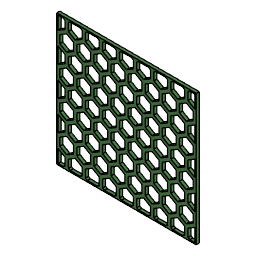
Rig (Autodesk Fusion 360 archive; units mm, degrees)
design "honey comb v1"
Autodesk Fusion 360 part; units mm, degrees
sketch "Sketch2" plane through (0, 0, 0) normal (0, 1, 0) x (1, 0, 0)
  line L0 (10, 5.7735) -> (0, 11.547)
  line L1 (0, 11.547) -> (-10, 5.7735)
  line L2 (-10, 5.7735) -> (-10, -5.7735)
  line L3 (-10, -5.7735) -> (0, -11.547)
  line L4 (0, -11.547) -> (10, -5.7735)
  line L5 (10, -5.7735) -> (10, 5.7735)
  line L6 (0, 0) -> (5, -8.6603) construction
  line L7 (-100, -94) -> (100, -94)
  line L8 (100, -94) -> (100, 94)
  line L9 (100, 94) -> (-100, 94)
  line L10 (-100, 94) -> (-100, -94)
  line L11 (-102, -96) -> (102, -96)
  line L12 (102, -96) -> (102, 96)
  line L13 (102, 96) -> (-102, 96)
  line L14 (-102, 96) -> (-102, -96)
  line L15 (0, -94) -> (0, -96) construction
  line L16 (100, 0) -> (102, 0) construction
  line L17 (-100, 0) -> (-102, 0) construction
  line L18 (0, 94) -> (0, 96) construction
  line L19 (-100, 0) -> (0, 0) construction
  line L20 (0, 0) -> (100, 0) construction
  dimension "d1" = 20
  dimension "d2" = 2
  dimension "d12" = 188
  dimension "d13" = 200
  constraint coincident L6.start L19.end
  constraint midpoint L4 L6.end
  constraint horizontal L7
  constraint perpendicular L7 L8
  constraint parallel L7 L9
  constraint parallel L8 L10
  constraint horizontal L11
  constraint vertical L12
  constraint horizontal L13
  constraint vertical L14
  constraint midpoint L7 L15.start
  constraint coincident L11 L15.end
  constraint perpendicular L11 L15
  constraint midpoint L8 L16.start
  constraint coincident L12 L16.end
  constraint perpendicular L12 L16
  constraint midpoint L10 L17.start
  constraint coincident L14 L17.end
  constraint perpendicular L14 L17
  constraint midpoint L9 L18.start
  constraint coincident L13 L18.end
  constraint perpendicular L13 L18
  constraint equal L15 L17
  constraint equal L17 L18
  constraint equal L16 L18
  constraint perpendicular L2 L19
  constraint perpendicular L8 L20
  constraint equal L19 L20
  measures "d1" distance of L2 L5
  measures "d2" distance of L7 L11
  measures "d12" distance of L7.end L8.end
  measures "d13" distance of L8.end L9.end
extrude "Extrude1" add sketch "Sketch2" against normal blind 10 contours L0 L1 L2 L3 L4 L5 | L7 L8 L9 L10
extrude "Extrude2" cut sketch "Sketch2" against normal through all contours L0 L1 L2 L3 L4 L5
pattern_linear "R-Pattern1" count 19 spacing 25 along (1, 0, 0) both ways count 19 spacing 25 along (0.5, 0, 0.866025) both ways of "Extrude2"
extrude "Extrude3" add sketch "Sketch2" against normal blind 10 contours L11 L12 L13 L14
extrude "Extrude4" cut 1 faces at (-75.8333, -10, -66.8764) along direction (0, 1, 0) blind 5.5
equation "d8 = d1 + 5 mm"
equation "d9 = d1 + 5 mm"

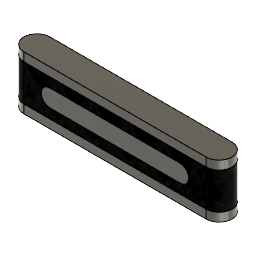
design "Conveyor Belt"
Autodesk Fusion 360 part; units mm, degrees
mirror "Mirror1" [no effect]
sketch "Sketch3" plane through (0, 0, 0) normal (0, 0, 1) x (1, 0, 0)
  line L0 (0, 0) -> (-525, 0)
  line L1 (-525, 0) -> (-525, -75)
  line L2 (-525, -75) -> (0, -75)
  line L3 (0, -75) -> (0, 0)
  circle A0 centre (-525, -37.5) radius 37.5
  circle A1 centre (0, -37.5) radius 37.5
  dimension "d12" = 75
  dimension "d13" = 525
  constraint horizontal L0
  constraint vertical L1
  constraint horizontal L2
  constraint vertical L3
  constraint coincident L0.start L3.end
  constraint coincident L0.end A0
  constraint tangent L0 A0
  constraint coincident L1.end A0
  measures "d12" distance of L0.start L2.end
  measures "d13" distance of L0.start L0.end
extrude "Extrude3" add sketch "Sketch3" along normal blind 155 makes body 1
sketch "Sketch4" plane through (0, -75, 0) normal (0, -1, 0) x (1, 0, 0)
  line L0 (-525, 0) -> (0, 0)
  line L1 (0, 0) -> (0, 155)
  line L2 (0, 155) -> (-525, 155)
  line L3 (-525, 155) -> (-525, 0)
  line L4 (-448.9835, 102.4793) -> (-75.0014, 102.5)
  line L5 (-448.9835, 52.5207) -> (-75.0014, 52.5)
  arc A0 (-448.9835, 102.4793) -> (-448.9835, 52.5207) centre (-450, 77.5) ccw
  arc A1 (-75.0014, 52.5) -> (-75.0014, 102.5) centre (-75, 77.5) ccw
  dimension "d16" = 50
  dimension "d17" = 75
  dimension "d18" = 50
  dimension "d19" = 75
  constraint tangent L4 A1
  constraint tangent L5 A1
  measures "d16" diameter of A0
  measures "d17" distance of L3 A0.centre
  measures "d18" diameter of A1
  measures "d19" distance of L1 A1.centre
extrude "Extrude4" add sketch "Sketch4" along normal blind 0.1 contours L4 L5 A0 A1 bodies 1
extrude "Extrude5" cut 1 faces at (-350, -50, 155) along direction (0, 0, -1) blind 130 on bodies 1 bodies 1 makes body 2 at (-350, -50, 0)
extrude "Extrude6" add 1 faces at (-350, -50, 25) along direction (0, 0, 1) blind 105 separate body on bodies 2 makes body 3
extrude "Extrude7" add 1 faces at (-350, -50, 130) along direction (0, 0, 1) blind 25 separate body on bodies 3 makes body 4
equation "d24 = 130.00 mm - 25 mm"

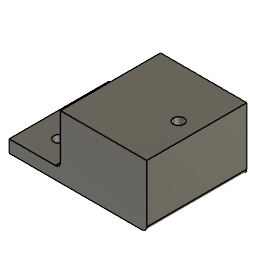
design "Rod Holder Thick"
Autodesk Fusion 360 part; units mm, degrees
sketch "Sketch1" plane through (0, 0, 0) normal (0, 0, 1) x (1, 0, 0)
  line L0 (0, 0) -> (55, 0)
  line L1 (55, 0) -> (55, 40)
  line L2 (55, 40) -> (0, 40)
  line L3 (0, 40) -> (0, 0)
  dimension "d1" = 55
  dimension "d2" = 40
  constraint horizontal L0
  constraint vertical L1
  constraint horizontal L2
  constraint vertical L3
  constraint coincident L0.start L3.end
  measures "d1" distance of L0.start L0.end
  measures "d2" distance of L0.start L2.end
extrude "Extrude1" add sketch "Sketch1" along normal blind 5
sketch "Sketch2" plane through (0, 0, 5) normal (0, 0, 1) x (-1, 0, 0)
  line L0 (0, -40) -> (0, 0)
  line L1 (0, 0) -> (-55, 0)
  line L2 (-55, 0) -> (-55, -40)
  line L3 (-55, -40) -> (0, -40)
  circle A0 centre (-10, -10) radius 2.15
  circle A1 centre (-10, -30) radius 2.15
  circle A2 centre (-47.75, -20) radius 2.15
  line L4 (-20.5, -40) -> (-20.5, 0)
  dimension "d5" = 4.3
  dimension "d6" = 4.3
  dimension "d7" = 20
  dimension "d8" = 10
  dimension "d9" = 10
  dimension "d10" = 4.3
  dimension "d11" = 7.25
  dimension "d12" = 20.5
  constraint coincident L3 L4.start
  constraint coincident L1 L4.end
  constraint perpendicular L1 L4
  measures "d5" diameter of A0
  measures "d6" diameter of A1
  measures "d7" distance of A0.centre A1.centre
  measures "d8" distance of L1 A0.centre
  measures "d9" distance of L0 A0.centre
  measures "d10" diameter of A2
  measures "d11" distance of L2 A2.centre
  measures "d12" distance of L0 L4
extrude "Extrude2" cut sketch "Sketch2" against normal blind 22 contours A0 | A1 | A2
extrude "Extrude3" add sketch "Sketch2" along normal blind 20 contours L1 L2 L3 L4
fillet "Fillet1" radius 2 1 edges at (20.5, 20, 5)
fillet "Fillet2" radius 2 1 edges at (55, 20, 0)

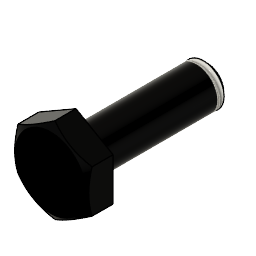
design "Hexagon Head Bolt DIN EN 24014 - M4 x 12 Steel 4.6 Black"
description: Hexagon Head Bolt DIN EN 24014 - M4 x 12
part number: DIN EN 24014 - M4 x 12 Steel 4.6 Black
Autodesk Fusion 360 part; units mm, degrees
sketch "Sketch1" plane through (0, 0, 0) normal (0, 1, 0) x (1, 0, 0)
  line L0 (-2, 0) -> (-2, 12)
  line L1 (-2, 12) -> (0, 12)
  line L2 (0, 12) -> (0, -2.8)
  line L3 (-2.94, -0.4) -> (-4.0425, -0.4)
  line L4 (-4.0425, -0.4) -> (-4.0425, -2.3858)
  line L5 (-2.94, -0.4) -> (-2.7091, 0)
  line L6 (-2.7091, 0) -> (-2, 0)
  line L7 (0, -2.8) -> (-3.325, -2.8)
  line L8 (-4.0425, -2.3858) -> (-3.325, -2.8)
  dimension "d81" = 8.085
  dimension "d123" = 0.4
  dimension "d127" = 12
  dimension "d149" = 4
  dimension "d157" = 30
  dimension "d158" = 6.65
  dimension "d162" = 2.8
  dimension "d163" = 30
  dimension "d164" = 5.88
  constraint perpendicular L0 L1
  constraint vertical L2
  constraint parallel L2 L4
  constraint coincident L2 L7.start
  constraint coincident origin L6
  constraint coincident L0.end L1.start
  constraint perpendicular L2 L7
  constraint coincident origin L2
  measures "d123" distance of L3 L6
  measures "d127" distance of L1 L6
  measures "d157" angle of L7 L8
  measures "d162" distance of L6 L7
  measures "d163" angle of L4 L5
revolve "Revolve1" add sketch "Sketch1" angle 360 about axis through (0, 0, -12) along (0, 0, 1)
sketch "Sketch8" plane through (0, 0, 0) normal (0, 0, 1) x (1, 0, 0)
  circle A0 centre (0, 0) radius 4.0425
  circle A1 centre (0, 0) radius 4.0425
  line L0 (-3.5009, -2.0213) -> (0, -4.0425)
  line L1 (0, -4.0425) -> (3.5009, -2.0212)
  line L2 (3.5009, -2.0212) -> (3.5009, 2.0213)
  line L3 (3.5009, 2.0213) -> (0, 4.0425)
  line L4 (0, 4.0425) -> (-3.5009, 2.0212)
  line L5 (-3.5009, 2.0212) -> (-3.5009, -2.0213)
  constraint coincident A1 L0.start
  constraint coincident A0.centre A1.centre
  constraint vertical L5
extrude "Extrude5" cut sketch "Sketch8" along normal through all contours A0 A1 L2 | A0 A1 L3 | A0 A1 L1 | A0 A1 L4 | A0 A1 L0 | A0 A1 L5
thread "Thread2" "ISO Metric profile 4.0 M4x0.7 M4x0.7 6g" major diameter 3.908 minor diameter 3.111 pitch 0.7 angle 60 resizes the face on face at (-1.9975, 0.0997, -8) from (0, 0, -11) to (0, 0, -12)
fillet "Fillet6" radius 0.2 1 edges at (1.954, 0, 0)
sketch "Sketch15" plane through (0, 0, 0) normal (0, 1, 0) x (1, 0, 0)
  line L0 (-2.04, 12) -> (-2.04, 11.5706)
  line L1 (-2.04, 11.5706) -> (-1.5706, 12)
  line L2 (0, 12) -> (0, -2.8)
  line L3 (-2.04, 12) -> (0, 12)
  dimension "d165" = 1.5706
  dimension "d166" = 2.04
  dimension "d167" = 0.4294
  constraint coincident L2.start L3.end
  constraint perpendicular L2 L3
  constraint coincident L1.end L3
  constraint perpendicular L0 L3
  measures "d165" distance of L1.end L2
  measures "d166" distance of L0 L2.start
  measures "d167" distance of L0.end L3
revolve "Revolve4" cut sketch "Sketch15" angle 360 about axis through (0, 0, 1.75) along (0, 0, 1)
equation "adsk_nomlen = 12.00 mm"
equation "adsk_headh = 2.80 mm"
equation "adsk_headdia = 8.085 mm"
equation "adsk_nomdia = 4.00 mm"
equation "d81 = adsk_headdia"
equation "adsk_waflat = 7.00 mm"
equation "adsk_thrlen = 1.00 mm"
equation "adsk_chamang2 = 30.00 deg"
equation "adsk_midfillet = 0.20 mm"
equation "d123 = adsk_necklen"
equation "adsk_necklen = 0.40 mm"
equation "adsk_neckdia = 5.88 mm"
equation "d127 = adsk_nomlen"
equation "d138 = adsk_midfillet"
equation "d140 = min(adsk_thrlen; adsk_nomlen - adsk_midfillet - 0.01 mm)"
equation "adsk_endpointdia = 3.14117 mm"
equation "adsk_startlen = 0.429415 mm"
equation "d149 = adsk_nomdia"
equation "d157 = adsk_chamang2"
equation "d158 = adsk_waflat * 0.95"
equation "adsk_neckang = 30 deg"
equation "d162 = adsk_headh"
equation "d163 = adsk_neckang"
equation "d164 = adsk_neckdia"
equation "d165 = adsk_endpointdia / 2"
equation "d166 = adsk_nomdia * 0.51"
equation "d167 = adsk_startlen"

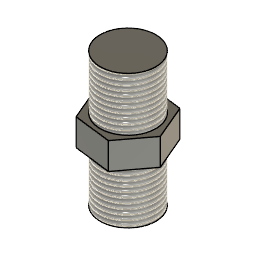
design "Male-Male Adaptor BSP"
Autodesk Fusion 360 part; units mm, degrees
sketch "Sketch1" plane through (0, 0, 0) normal (0, 0, 1) x (1, 0, 0)
  circle A0 centre (0, 0) radius 10
  dimension "d1" = 20
  constraint coincident A0.centre origin
  measures "d1" diameter of A0
extrude "Extrude1" add sketch "Sketch1" along normal blind 20
sketch "Sketch2" plane through (0, 0, 20) normal (0, 0, 1) x (-1, 0, 0)
  circle A0 centre (0, 0) radius 10
  line L0 (-8.3368, -11.0679) -> (5.4167, -12.7538)
  line L1 (5.4167, -12.7538) -> (13.7535, -1.6859)
  line L2 (13.7535, -1.6859) -> (8.3368, 11.0679)
  line L3 (8.3368, 11.0679) -> (-5.4167, 12.7538)
  line L4 (-5.4167, 12.7538) -> (-13.7535, 1.6859)
  line L5 (-13.7535, 1.6859) -> (-8.3368, -11.0679)
  dimension "d4" = 12
  constraint coincident A0.centre origin
  measures "d4" distance of A0.centre L5
extrude "Extrude2" add sketch "Sketch2" along normal blind 10 contours A0 | L0 L1 L2 L3 L4 L5
sketch "Sketch3" plane through (0, 0, 30) normal (0, 0, 1) x (-1, 0, 0)
  line L0 (-13.7535, 1.6859) -> (-8.3368, -11.0679)
  line L1 (-8.3368, -11.0679) -> (5.4167, -12.7538)
  line L2 (5.4167, -12.7538) -> (13.7535, -1.6859)
  line L3 (13.7535, -1.6859) -> (8.3368, 11.0679)
  line L4 (8.3368, 11.0679) -> (-5.4167, 12.7538)
  line L5 (-5.4167, 12.7538) -> (-13.7535, 1.6859)
  circle A0 centre (0, 0) radius 10
  dimension "d7" = 20
  constraint coincident A0.centre origin
  measures "d7" diameter of A0
extrude "Extrude3" add sketch "Sketch3" along normal blind 20 contours A0
thread "Thread1" "BSP Pipe Threads 1/2 G 1/2-14 G 1/2-14" major diameter 20.813 minor diameter 18.631 pitch 1.8143 angle 55 resizes the face on face at (9.9876, -0.4985, 13.3333) on face at (-9.9876, 0.4985, 43.3333)

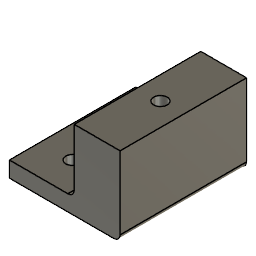
design "Rod Holding Bracket"
Autodesk Fusion 360 part; units mm, degrees
sketch "Sketch1" plane through (0, 0, 0) normal (0, 0, 1) x (1, 0, 0)
  line L0 (0, 0) -> (35, 0)
  line L1 (35, 0) -> (35, 40)
  line L2 (35, 40) -> (0, 40)
  line L3 (0, 40) -> (0, 0)
  dimension "d1" = 35
  dimension "d2" = 40
  constraint horizontal L0
  constraint vertical L1
  constraint horizontal L2
  constraint vertical L3
  constraint coincident L0.start L3.end
  measures "d1" distance of L0.start L0.end
  measures "d2" distance of L0.start L2.end
extrude "Extrude1" add sketch "Sketch1" along normal blind 5
sketch "Sketch2" plane through (0, 0, 5) normal (0, 0, 1) x (-1, 0, 0)
  line L0 (0, -40) -> (0, 0)
  line L1 (0, 0) -> (-35, 0)
  line L2 (-35, 0) -> (-35, -40)
  line L3 (-35, -40) -> (0, -40)
  circle A0 centre (-10, -10) radius 2.15
  circle A1 centre (-10, -30) radius 2.15
  circle A2 centre (-27.75, -20) radius 2.15
  line L4 (-20.5, -40) -> (-20.5, 0)
  dimension "d5" = 4.3
  dimension "d6" = 4.3
  dimension "d7" = 20
  dimension "d8" = 10
  dimension "d9" = 10
  dimension "d10" = 4.3
  dimension "d11" = 7.25
  dimension "d12" = 20.5
  constraint coincident L3 L4.start
  constraint coincident L1 L4.end
  constraint perpendicular L1 L4
  measures "d5" diameter of A0
  measures "d6" diameter of A1
  measures "d7" distance of A0.centre A1.centre
  measures "d8" distance of L1 A0.centre
  measures "d9" distance of L0 A0.centre
  measures "d10" diameter of A2
  measures "d11" distance of L2 A2.centre
  measures "d12" distance of L0 L4
extrude "Extrude2" cut sketch "Sketch2" against normal blind 22 contours A0 | A1 | A2
extrude "Extrude3" add sketch "Sketch2" along normal blind 20 contours L1 L2 L3 L4
fillet "Fillet1" radius 2 1 edges at (20.5, 20, 5)
fillet "Fillet2" radius 2 1 edges at (35, 20, 0)

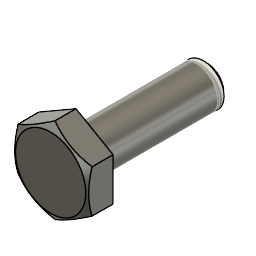
design "Hexagon Head Bolt DIN EN 24014 - M4 x 12 Steel 4.6 Plain"
description: Hexagon Head Bolt DIN EN 24014 - M4 x 12
part number: DIN EN 24014 - M4 x 12 Steel 4.6 Plain
Autodesk Fusion 360 part; units mm, degrees
sketch "Sketch1" plane through (0, 0, 0) normal (0, 1, 0) x (1, 0, 0)
  line L0 (-2, 0) -> (-2, 12)
  line L1 (-2, 12) -> (0, 12)
  line L2 (0, 12) -> (0, -2.8)
  line L3 (-2.94, -0.4) -> (-4.0425, -0.4)
  line L4 (-4.0425, -0.4) -> (-4.0425, -2.3858)
  line L5 (-2.94, -0.4) -> (-2.7091, 0)
  line L6 (-2.7091, 0) -> (-2, 0)
  line L7 (0, -2.8) -> (-3.325, -2.8)
  line L8 (-4.0425, -2.3858) -> (-3.325, -2.8)
  dimension "d81" = 8.085
  dimension "d123" = 0.4
  dimension "d127" = 12
  dimension "d149" = 4
  dimension "d157" = 30
  dimension "d158" = 6.65
  dimension "d162" = 2.8
  dimension "d163" = 30
  dimension "d164" = 5.88
  constraint perpendicular L0 L1
  constraint vertical L2
  constraint parallel L2 L4
  constraint coincident L2 L7.start
  constraint coincident origin L6
  constraint coincident L0.end L1.start
  constraint perpendicular L2 L7
  constraint coincident origin L2
  measures "d123" distance of L3 L6
  measures "d127" distance of L1 L6
  measures "d157" angle of L7 L8
  measures "d162" distance of L6 L7
  measures "d163" angle of L4 L5
revolve "Revolve1" add sketch "Sketch1" angle 360 about axis through (0, 0, -12) along (0, 0, 1)
sketch "Sketch8" plane through (0, 0, 0) normal (0, 0, 1) x (1, 0, 0)
  circle A0 centre (0, 0) radius 4.0425
  circle A1 centre (0, 0) radius 4.0425
  line L0 (-3.5009, -2.0213) -> (0, -4.0425)
  line L1 (0, -4.0425) -> (3.5009, -2.0212)
  line L2 (3.5009, -2.0212) -> (3.5009, 2.0213)
  line L3 (3.5009, 2.0213) -> (0, 4.0425)
  line L4 (0, 4.0425) -> (-3.5009, 2.0212)
  line L5 (-3.5009, 2.0212) -> (-3.5009, -2.0213)
  constraint coincident A1 L0.start
  constraint coincident A0.centre A1.centre
  constraint vertical L5
extrude "Extrude5" cut sketch "Sketch8" along normal through all contours A0 A1 L2 | A0 A1 L3 | A0 A1 L1 | A0 A1 L4 | A0 A1 L0 | A0 A1 L5
thread "Thread2" "ISO Metric profile 4.0 M4x0.7 M4x0.7 6g" major diameter 3.908 minor diameter 3.111 pitch 0.7 angle 60 resizes the face on face at (-1.9901, 0.1991, -8) from (0, 0, -11) to (0, 0, -12)
fillet "Fillet6" radius 0.2 1 edges at (1.954, 0, 0)
sketch "Sketch15" plane through (0, 0, 0) normal (0, 1, 0) x (1, 0, 0)
  line L0 (-2.04, 12) -> (-2.04, 11.5706)
  line L1 (-2.04, 11.5706) -> (-1.5706, 12)
  line L2 (0, 12) -> (0, -2.8)
  line L3 (-2.04, 12) -> (0, 12)
  dimension "d165" = 1.5706
  dimension "d166" = 2.04
  dimension "d167" = 0.4294
  constraint coincident L2.start L3.end
  constraint perpendicular L2 L3
  constraint coincident L1.end L3
  constraint perpendicular L0 L3
  measures "d165" distance of L1.end L2
  measures "d166" distance of L0 L2.start
  measures "d167" distance of L0.end L3
revolve "Revolve4" cut sketch "Sketch15" angle 360 about axis through (0, 0, 1.75) along (0, 0, 1)
equation "adsk_nomlen = 12.00 mm"
equation "adsk_headh = 2.80 mm"
equation "adsk_headdia = 8.085 mm"
equation "adsk_nomdia = 4.00 mm"
equation "d81 = adsk_headdia"
equation "adsk_waflat = 7.00 mm"
equation "adsk_thrlen = 1.00 mm"
equation "adsk_chamang2 = 30.00 deg"
equation "adsk_midfillet = 0.20 mm"
equation "d123 = adsk_necklen"
equation "adsk_necklen = 0.40 mm"
equation "adsk_neckdia = 5.88 mm"
equation "d127 = adsk_nomlen"
equation "d138 = adsk_midfillet"
equation "d140 = min(adsk_thrlen; adsk_nomlen - adsk_midfillet - 0.01 mm)"
equation "adsk_endpointdia = 3.14117 mm"
equation "adsk_startlen = 0.429415 mm"
equation "d149 = adsk_nomdia"
equation "d157 = adsk_chamang2"
equation "d158 = adsk_waflat * 0.95"
equation "adsk_neckang = 30 deg"
equation "d162 = adsk_headh"
equation "d163 = adsk_neckang"
equation "d164 = adsk_neckdia"
equation "d165 = adsk_endpointdia / 2"
equation "d166 = adsk_nomdia * 0.51"
equation "d167 = adsk_startlen"

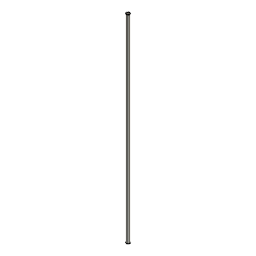
design "M4 Threaded Sliding Rod"
Autodesk Fusion 360 part; units mm, degrees
sketch "Sketch1" plane through (0, 0, 0) normal (0, 0, 1) x (1, 0, 0)
  circle A0 centre (0, 0) radius 2.15
  dimension "d1" = 4.3
  constraint coincident A0.centre origin
  measures "d1" diameter of A0
extrude "Extrude1" add sketch "Sketch1" along normal blind 250

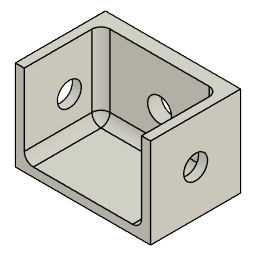
design "Alternate 3 Way Bracket 30x20x20"
Autodesk Fusion 360 part; units mm, degrees
sketch "Sketch1" plane through (0, 0, 0) normal (0, 0, 1) x (1, 0, 0)
  line L0 (0, 0) -> (30, 0)
  line L1 (30, 0) -> (30, 20)
  line L2 (30, 20) -> (0, 20)
  line L3 (0, 20) -> (0, 0)
  dimension "d1" = 20
  dimension "d2" = 30
  constraint horizontal L0
  constraint vertical L1
  constraint horizontal L2
  constraint vertical L3
  constraint coincident L0.start L3.end
  measures "d1" distance of L0.start L2.end
  measures "d2" distance of L0.start L0.end
extrude "Extrude1" add sketch "Sketch1" along normal blind 2
sketch "Sketch2" plane through (0, 0, 2) normal (0, 0, 1) x (-1, 0, 0)
  line L0 (0, -20) -> (0, 0)
  line L1 (0, 0) -> (-30, 0)
  line L2 (-30, 0) -> (-30, -20)
  line L3 (-30, -20) -> (0, -20)
  line L4 (0, 0) -> (-2, 0) construction
  line L5 (-2, 0) -> (-2, -17)
  line L6 (-2, -17) -> (-28, -17)
  line L7 (-28, -17) -> (-28, 0)
  line L8 (-28, 0) -> (-30, 0) construction
  line L9 (-15, -20) -> (-15, 0) construction
  line L10 (0, -20) -> (0, 0)
  line L11 (-30, -20) -> (0, -20)
  dimension "d27" = 2
  dimension "d28" = 3
  constraint coincident L0.end L1.start
  constraint coincident L1 L4.end
  constraint perpendicular L3 L5
  constraint perpendicular L5 L6
  constraint coincident L1 L7.end
  constraint perpendicular L1 L7
  constraint coincident L1.end L2.start
  constraint midpoint L3 L9.start
  constraint midpoint L1 L9.end
  constraint symmetric L5 L7 L9
  measures "d27" distance of L5 L10
  measures "d28" distance of L6 L11
extrude "Extrude2" add sketch "Sketch2" along normal blind 18 contours L0 L1 L2 L3 L5 L6 L7 L10 L11
sketch "Sketch5" plane through (0, 20, 0) normal (0, 1, 0) x (-1, 0, 0)
  line L0 (-30, 0) -> (0, 0)
  line L1 (0, 0) -> (0, 20)
  line L2 (0, 20) -> (-30, 20)
  line L3 (-30, 20) -> (-30, 0)
  circle A0 centre (-15, 10) radius 2.65
  line L4 (-15, 20) -> (-15, 0) construction
  dimension "d15" = 5.3
  constraint midpoint L2 L4.start
  constraint midpoint L0 L4.end
  constraint midpoint A0.centre L4
  measures "d15" diameter of A0
sketch "Sketch6" plane through (0, 0, 0) normal (-1, 0, 0) x (0, -1, 0)
  line L0 (-20, 0) -> (0, 0)
  line L1 (0, 0) -> (0, 20)
  line L2 (0, 20) -> (-20, 20)
  line L3 (-20, 20) -> (-20, 0)
  circle A0 centre (-10, 10) radius 2.65
  dimension "d16" = 5.3
  measures "d16" diameter of A0
extrude "Extrude5" cut sketch "Sketch6" against normal blind 30 contours A0
extrude "Extrude6" cut sketch "Sketch5" against normal blind 4 contours A0
fillet "Fillet1" radius 2 1 edges at (2, 17, 11)
fillet "Fillet2" radius 2 1 edges at (28, 17, 11)
fillet "Fillet3" radius 2 5 edges at (28, 7.5, 2) (27.4142, 16.4142, 2) (15, 17, 2) (2.5858, 16.4142, 2) (2, 7.5, 2)

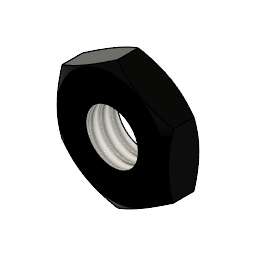
design "Hexagon Nut BS 4183 - M4 Steel 6 Black"
description: Hexagon Nut BS 4183 - M4
part number: HN BS 4183 - M4 Steel 6 Black
Autodesk Fusion 360 part; units mm, degrees
sketch "Sketch1" plane through (0, 0, 0) normal (0, 1, 0) x (1, 0, 0)
  line L0 (0, 0) -> (0, -2)
  line L1 (-2, 0) -> (-3.43, 0)
  line L2 (-3.43, 0) -> (-4.0425, -0.3536)
  line L3 (-4.0425, -0.3536) -> (-4.0425, -1.6464)
  line L4 (-4.0425, -1.6464) -> (-3.43, -2)
  line L5 (-3.43, -2) -> (-2, -2)
  line L6 (-2, -2) -> (-2, 0)
  dimension "d121" = 4
  dimension "d122" = 30
  dimension "d123" = 30
  dimension "d125" = 6.86
  dimension "d128" = 8.085
  dimension "d153" = 2
  constraint vertical L0
  constraint coincident L0 L0.end
  constraint coincident origin L0
  constraint coincident L0.start L1
  constraint coincident L0.start origin
  constraint vertical L1.end L4.end
  constraint coincident L0.end L5
  constraint horizontal L1
  measures "d122" angle of L1 L2
  measures "d123" angle of L4 L5
  measures "d153" distance of L1 L5
revolve "Revolve1" add sketch "Sketch1" angle 360 about axis through (0, 0, 0) along (0, 0, 1)
sketch "Sketch8" plane through (0, 0, 2) normal (0, 0, 1) x (1, 0, 0)
  line L0 (-3.5, -2.0228) -> (-3.5, 2.0228)
  circle A0 centre (0, 0) radius 2
  circle A1 centre (0, 0) radius 4.0425
  dimension "d114" = 3.5
  constraint coincident L0.end A1
  constraint coincident L0.start A1
  constraint vertical L0
  measures "d114" distance of A0.centre L0
extrude "Extrude5" cut sketch "Sketch8" against normal blind 2 contours L0 A1 picked at (-3.5875, 0.4927)
pattern_circular "C-Pattern2" count 6 over 360 about axis through (0, 0, 1.75) along (0, 0, 1) of "Extrude5"
thread "Thread3" "ISO Metric profile 4.0 M4x0.7 M4x0.7 6H" major diameter 4.1095 minor diameter 3.332 pitch 0.7 angle 60 resizes the face on face at (-1.9901, 0.1991, 1.3333)
equation "adsk_nheig = 2.00 mm"
equation "adsk_maxdia = 8.085 mm"
equation "adsk_nomdia = 4.00 mm"
equation "d89 = -adsk_nheig"
equation "adsk_waflat = 7.00 mm"
equation "d114 = adsk_waflat / 2"
equation "adsk_chamang1 = 30 deg"
equation "adsk_chamang2 = 30 deg"
equation "d121 = adsk_nomdia"
equation "d122 = adsk_chamang1"
equation "d123 = adsk_chamang2"
equation "d125 = adsk_beardia"
equation "d128 = adsk_maxdia"
equation "d147 = adsk_nheig"
equation "adsk_beardia = adsk_waflat * 0.98"
equation "d153 = adsk_nheig"

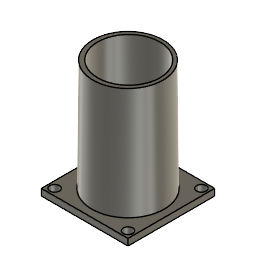
design "28ID32OD"
Autodesk Fusion 360 part; units mm, degrees
sketch "Sketch1" plane through (0, 0, 0) normal (0, 0, 1) x (1, 0, 0)
  line L0 (19.5, 19.5) -> (-19.5, 19.5)
  line L1 (-19.5, 19.5) -> (-19.5, -19.5)
  line L2 (-19.5, -19.5) -> (19.5, -19.5)
  line L3 (19.5, -19.5) -> (19.5, 19.5)
  line L4 (19.5, 19.5) -> (-19.5, -19.5) construction
  line L5 (-19.5, 19.5) -> (19.5, -19.5) construction
  circle A0 centre (-16.5, 16.5) radius 2.15
  line L6 (0, 19.5) -> (0, -19.5) construction
  line L7 (-19.5, 0) -> (19.5, 0) construction
  circle A1 centre (-16.5, -16.5) radius 2.15
  circle A2 centre (16.5, 16.5) radius 2.15
  circle A3 centre (16.5, -16.5) radius 2.15
  dimension "d1" = 39
  dimension "d2" = 39
  dimension "d3" = 4.3
  dimension "d4" = 3
  constraint horizontal L0
  constraint perpendicular L0 L1
  constraint parallel L0 L2
  constraint parallel L1 L3
  constraint coincident L4 origin
  constraint coincident L5 origin
  constraint coincident L5 A0.centre
  constraint midpoint L0 L6.start
  constraint midpoint L2 L6.end
  constraint midpoint L1 L7.start
  constraint midpoint L3 L7.end
  constraint symmetric A0 L7 A1
  constraint symmetric A0 L6 A2
  constraint symmetric L6 A1 A3
  measures "d1" distance of L0.start L0.end
  measures "d2" distance of L0.start L2.end
  measures "d3" diameter of A0
  measures "d4" distance of L0 A0.centre
extrude "Extrude1" add sketch "Sketch1" along normal blind 3
sketch "Sketch2" plane through (0, 0, 3) normal (0, 0, 1) x (-1, 0, 0)
  circle A0 centre (16.5, -16.5) radius 2.15
  circle A1 centre (-16.5, 16.5) radius 2.15
  circle A2 centre (-16.5, -16.5) radius 2.15
  circle A3 centre (16.5, 16.5) radius 2.15
  line L0 (-19.5, 19.5) -> (-19.5, -19.5)
  line L1 (-19.5, -19.5) -> (19.5, -19.5)
  line L2 (19.5, -19.5) -> (19.5, 19.5)
  line L3 (19.5, 19.5) -> (-19.5, 19.5)
  circle A4 centre (0, 0) radius 16.25
  dimension "d7" = 32.5
  constraint coincident A4.centre origin
  measures "d7" diameter of A4
ref_plane "WorkPlane1" through (0, 0, 53) normal (0, 0, 1) x (-1, 0, 0)
sketch "Sketch3" plane through (0, 0, 53) normal (0, 0, 1) x (1, 0, 0)
  circle A0 centre (0, 0) radius 15.75
  dimension "d9" = 31.5
  constraint coincident A0.centre origin
  measures "d9" diameter of A0
loft "Loft1" add profiles "Sketch2", "Sketch3" section 1 contours A4 section 2
hole "Hole1" at (0.1469, 0.2089, 53) direction (0, 0, -1) diameter 28 depth 55 tip angle 118

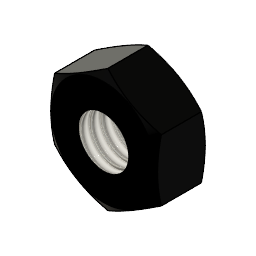
design "Hex Nut Style 1 ANSI B18.2.4.1M - M4 Steel Grade 2H Black"
description: Hex Nut Style 1 ANSI B18.2.4.1M - M4
part number: HNS1 ANSI B18.2.4.1M - M4 Steel Grade 2H Black
Autodesk Fusion 360 part; units mm, degrees
sketch "Sketch1" plane through (0, 0, 0) normal (0, 1, 0) x (1, 0, 0)
  line L0 (0, 0) -> (0, -3.2)
  line L1 (-2, 0) -> (-3.43, 0)
  line L2 (-3.43, 0) -> (-4.0425, -0.2856)
  line L3 (-4.0425, -0.2856) -> (-4.0425, -2.9144)
  line L4 (-4.0425, -2.9144) -> (-3.43, -3.2)
  line L5 (-3.43, -3.2) -> (-2, -3.2)
  line L6 (-2, -3.2) -> (-2, 0)
  dimension "d121" = 4
  dimension "d122" = 25
  dimension "d123" = 25
  dimension "d125" = 6.86
  dimension "d128" = 8.085
  dimension "d153" = 3.2
  constraint vertical L0
  constraint coincident L0 L0.end
  constraint coincident origin L0
  constraint coincident L0.start L1
  constraint coincident L0.start origin
  constraint vertical L1.end L4.end
  constraint coincident L0.end L5
  constraint horizontal L1
  measures "d122" angle of L1 L2
  measures "d123" angle of L4 L5
  measures "d153" distance of L1 L5
revolve "Revolve1" add sketch "Sketch1" angle 360 about axis through (0, 0, 0) along (0, 0, 1)
sketch "Sketch8" plane through (0, 0, 3.2) normal (0, 0, 1) x (1, 0, 0)
  line L0 (-3.5, -2.0228) -> (-3.5, 2.0228)
  circle A0 centre (0, 0) radius 2
  circle A1 centre (0, 0) radius 4.0425
  dimension "d114" = 3.5
  constraint coincident L0.end A1
  constraint coincident L0.start A1
  constraint vertical L0
  measures "d114" distance of A0.centre L0
extrude "Extrude5" cut sketch "Sketch8" against normal blind 3.2 contours L0 A1 picked at (-3.5875, 0.4927)
pattern_circular "C-Pattern2" count 6 over 360 about axis through (0, 0, 1.75) along (0, 0, 1) of "Extrude5"
thread "Thread3" "ANSI Metric M Profile 4.0 M4x0.7 M4x0.7 6H" major diameter 4.1095 minor diameter 3.332 pitch 0.7 angle 60 resizes the face on face at (-1.9975, 0.0997, 2.1333)
equation "adsk_nheig = 3.20 mm"
equation "adsk_maxdia = 8.085 mm"
equation "adsk_nomdia = 4.00 mm"
equation "d89 = -adsk_nheig"
equation "adsk_waflat = 7.00 mm"
equation "d114 = adsk_waflat / 2"
equation "adsk_chamang1 = 25.00 deg"
equation "adsk_chamang2 = 25.00 deg"
equation "d121 = adsk_nomdia"
equation "d122 = adsk_chamang1"
equation "d123 = adsk_chamang2"
equation "d125 = adsk_beardia"
equation "d128 = adsk_maxdia"
equation "d147 = adsk_nheig"
equation "adsk_beardia = adsk_waflat * 0.98"
equation "d153 = adsk_nheig"

design "Hex Bolt ANSI B18.2.3.5M - M5 x 0.8 x 10 Steel Grade 2 Black"
description: Hex Bolt ANSI B18.2.3.5M - M5 x 0.8 x 10
part number: HH ANSI B18.2.3.5M - M5 x 0.8 x 10 Steel Grade 2 Black
Autodesk Fusion 360 part; units mm, degrees
sketch "Sketch1" plane through (0, 0, 0) normal (0, 1, 0) x (1, 0, 0)
  line L0 (-2.5, 0) -> (-2.5, 10)
  line L1 (-2.5, 10) -> (0, 10)
  line L2 (0, 10) -> (0, -3.58)
  line L3 (-2.5, 0) -> (-4.62, 0)
  line L4 (-4.62, 0) -> (-4.62, -3.1759)
  line L5 (-3.92, -3.58) -> (0, -3.58)
  line L6 (-4.62, -3.1759) -> (-3.92, -3.58)
  dimension "d81" = 9.24
  dimension "d135" = 5
  dimension "d139" = 3.58
  dimension "d140" = 10
  dimension "d156" = 7.84
  dimension "d158" = 30
  constraint perpendicular L0 L1
  constraint collinear origin L1.end L2.end
  constraint perpendicular L0 L3
  constraint coincident origin L3
  constraint vertical L2
  constraint coincident L2 L5.end
  constraint coincident L0.start L3.start
  constraint coincident L0.end L1.start
  constraint vertical L4
  measures "d139" distance of L3 L5
  measures "d140" distance of L1 L3
  measures "d158" angle of L5 L6
revolve "Revolve1" add sketch "Sketch1" angle 360 about axis through (0, 0, -10) along (0, 0, 1)
sketch "Sketch8" plane through (0, 0, 3.58) normal (0, 0, 1) x (1, 0, 0)
  circle A0 centre (0, 0) radius 4.62
  line L0 (-4.001, -2.31) -> (0, -4.62)
  line L1 (0, -4.62) -> (4.001, -2.31)
  line L2 (4.001, -2.31) -> (4.001, 2.31)
  line L3 (4.001, 2.31) -> (0, 4.62)
  line L4 (0, 4.62) -> (-4.001, 2.31)
  line L5 (-4.001, 2.31) -> (-4.001, -2.31)
  constraint coincident A0 L0.start
  constraint coincident A0.centre origin
  constraint vertical L5
extrude "Extrude5" cut sketch "Sketch8" against normal blind 3.58 contours A0 L2 | A0 L3 | A0 L1 | A0 L4 | A0 L0 | A0 L5
fillet "Fillet7" radius 0.2 1 edges at (-2.3308, 0.904, 0)
thread "Thread4" "ANSI Metric M Profile 5.0 M5x0.8 M5x0.8 6g" major diameter 4.901 minor diameter 3.9895 pitch 0.8 angle 60 resizes the face on face at (-2.4876, 0.2489, -6.7333) from (0, 0, -2) to (0, 0, -10)
sketch "Sketch13" plane through (0, 0, 0) normal (0, 1, 0) x (1, 0, 0)
  line L0 (0, 10) -> (0, -3.58) construction
  line L1 (0, 10) -> (-2.55, 10)
  line L2 (-2.55, 10) -> (-2.55, 9.5092)
  line L3 (-2.55, 9.5092) -> (-2.0092, 10)
  dimension "d160" = 0.4908
  dimension "d161" = 2.0092
  dimension "d162" = 2.55
  constraint coincident L0.start L1.start
  constraint perpendicular L0 L1
  constraint perpendicular L1 L2
  constraint coincident L1 L3.end
  measures "d160" distance of L1 L2.end
  measures "d161" distance of L0 L3.end
  measures "d162" distance of L0.start L2
revolve "Revolve4" cut sketch "Sketch13" angle 360 about axis through (0, 0, 1.75) along (0, 0, 1)
equation "adsk_nomlen = 10.00 mm"
equation "adsk_headh = 3.58 mm"
equation "adsk_headdia = 9.24 mm"
equation "adsk_nomdia = 5.00 mm"
equation "d81 = adsk_headdia"
equation "d89 = -adsk_headh"
equation "adsk_waflat = 8.00 mm"
equation "adsk_thrlen = 8.00 mm"
equation "adsk_midfillet = 0.20 mm"
equation "d135 = adsk_nomdia"
equation "d139 = adsk_headh"
equation "d140 = adsk_nomlen"
equation "d142 = adsk_midfillet"
equation "adsk_endpointdia = 4.01848 mm"
equation "adsk_startlen = 0.49076 mm"
equation "d156 = adsk_waflat * 0.98"
equation "d158 = adsk_chamang2"
equation "adsk_chamang2 = 30.00 deg"
equation "d160 = adsk_startlen"
equation "d161 = adsk_endpointdia / 2"
equation "d162 = adsk_nomdia * 0.51"
equation "d166 = min(adsk_thrlen; adsk_nomlen - adsk_midfillet - 0.001 mm)"

design "Needle Valve Placeholder"
Autodesk Fusion 360 part; units mm, degrees
sketch "Sketch1" plane through (0, 0, 0) normal (0, 0, 1) x (1, 0, 0)
  line L0 (0, 0) -> (27, 0)
  line L1 (27, 0) -> (27, 27)
  line L2 (27, 27) -> (0, 27)
  line L3 (0, 27) -> (0, 0)
  dimension "d1" = 27
  dimension "d2" = 27
  constraint horizontal L0
  constraint vertical L1
  constraint horizontal L2
  constraint vertical L3
  constraint coincident L0.start L3.end
  measures "d1" distance of L0.start L2.end
  measures "d2" distance of L0.start L0.end
extrude "Extrude1" add sketch "Sketch1" along normal blind 27
sketch "Sketch2" plane through (0, 0, 0) normal (0, -1, 0) x (1, 0, 0)
  line L0 (0, 0) -> (27, 0)
  line L1 (27, 0) -> (27, 27)
  line L2 (27, 27) -> (0, 27)
  line L3 (0, 27) -> (0, 0)
  circle A0 centre (13.5, 13.5) radius 13
  circle A1 centre (13.5, 13.5) radius 9.9247
  dimension "d5" = 26
  constraint concentric A0 A1
  measures "d5" diameter of A0
extrude "Extrude2" add sketch "Sketch2" along normal blind 12 contours A0
ref_plane "WorkPlane1" through (13.5, 13.5, 13.5) normal (0, -1, 0) x (1, 0, 0)
mirror "Mirror1" about plane through (13.5, 13.5, 13.5) normal (0, -1, 0) of "Extrude2"
thread "Thread1" "BSP Pipe Threads 1/2 G 1/2-14 G 1/2-14" major diameter 20.955 minor diameter 18.9015 pitch 1.8143 angle 55 resizes the face on face at (23.4124, -8, 13.0053) on face at (23.4124, 35, 13.0053)
sketch "Sketch3" plane through (0, 0, 27) normal (0, 0, 1) x (-1, 0, 0)
  line L0 (0, -27) -> (0, 0)
  line L1 (0, 0) -> (-27, 0)
  line L2 (-27, 0) -> (-27, -27)
  line L3 (-27, -27) -> (0, -27)
  circle A0 centre (-13.5, -13.5) radius 6.75
  dimension "d12" = 13.5
  measures "d12" diameter of A0
extrude "Extrude3" add sketch "Sketch3" along normal blind 50 contours A0
sketch "Sketch4" plane through (0, 0, 77) normal (0, 0, 1) x (-1, 0, 0)
  circle A0 centre (-13.5, -13.5) radius 6.75
  circle A1 centre (-13.5, -13.5) radius 13.5
  dimension "d15" = 27
  constraint concentric A0 A1
  measures "d15" diameter of A1
extrude "Extrude4" add sketch "Sketch4" along normal blind 8 contours A0 | A1
